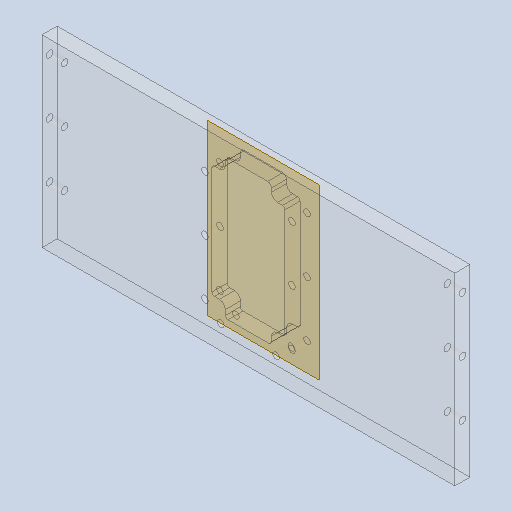
# Autodesk Inventor part: _newbody1
Saved by Autodesk Inventor 2024.3 (Build 283343000, 343)
## iProperties
Created: 2024-09-09
Part Number: _newbody1
Material: PMMA 플라스틱
Document SubType Name: Modeling
Designer: gretc
Density: 1.188 g/cm^3
Appearance: 폴리카보네이트 - 선명
Author: gretc
Autodesk Inventor part; units mm, degrees
ref_plane "YZ Plane" through (0, 0, 0) normal (1, 0, 0) x (0, 1, 0)
ref_plane "XZ Plane" through (0, 0, 0) normal (0, 1, 0) x (-1, 0, 0)
ref_plane "XY Plane" through (0, 0, 0) normal (0, 0, 1) x (1, 0, 0)
ref_plane "작업 평면1" through (0, 0, 0) normal (0, 0, 1) x (1, 0, 0)
ref_plane "작업 평면2" through (0, 0, 0) normal (0, 0, 1) x (1, 0, 0)
sketch "스케치2" plane through (0, 0, 0) normal (0, 0, 1) x (1, 0, 0)
  arc A0 (20.1, 4.5766) -> (19.5808, 6.2636) centre (17.1, 4.5766) ccw projected
  line L0 (20.1, -39.6766) -> (20.1, 4.5766) projected
  arc A1 (19.5808, -41.3636) -> (20.1, -39.6766) centre (17.1, -39.6766) ccw projected
  line L1 (15.8929, -46.7869) -> (19.5808, -41.3636) projected
  arc A2 (13.4121, -48.1) -> (15.8929, -46.7869) centre (13.4121, -45.1) ccw projected
  line L2 (-13.4121, -48.1) -> (13.4121, -48.1) projected
  arc A3 (-15.8929, -46.7869) -> (-13.4121, -48.1) centre (-13.4121, -45.1) ccw projected
  line L3 (-19.5808, -41.3636) -> (-15.8929, -46.7869) projected
  arc A4 (-20.1, -39.6766) -> (-19.5808, -41.3636) centre (-17.1, -39.6766) ccw projected
  line L4 (-20.1, 4.5766) -> (-20.1, -39.6766) projected
  arc A5 (-19.5808, 6.2636) -> (-20.1, 4.5766) centre (-17.1, 4.5766) ccw projected
  line L5 (-15.5953, 12.1246) -> (-19.5808, 6.2636) projected
  arc A6 (-13.9414, 13) -> (-15.5953, 12.1246) centre (-13.9414, 11) ccw projected
  line L6 (-7.65, 13) -> (-13.9414, 13) projected
  arc A7 (-7.65, 13) -> (-9.15, 11.5) centre (-7.65, 11.5) ccw projected
  line L7 (-9.15, 11.5) -> (-9.15, 10) projected
  arc A8 (-11.5, 7.65) -> (-9.15, 10) centre (-11.5, 10) ccw projected
  line L8 (-11.5, 7.65) -> (-13.5, 7.65) projected
  arc A9 (-13.5, 7.65) -> (-14.5, 6.65) centre (-13.5, 6.65) ccw projected
  line L9 (-14.5, 6.65) -> (-14.5, -36.15) projected
  arc A10 (-14.5, -36.15) -> (-13.5, -37.15) centre (-13.5, -36.15) ccw projected
  line L10 (-13.5, -37.15) -> (-11.5, -37.15) projected
  arc A11 (-9.15, -39.5) -> (-11.5, -37.15) centre (-11.5, -39.5) ccw projected
  line L11 (-9.15, -39.5) -> (-9.15, -41.5) projected
  arc A12 (-9.15, -41.5) -> (-8.15, -42.5) centre (-8.15, -41.5) ccw projected
  line L12 (-8.15, -42.5) -> (8.15, -42.5) projected
  arc A13 (8.15, -42.5) -> (9.15, -41.5) centre (8.15, -41.5) ccw projected
  line L13 (9.15, -41.5) -> (9.15, -39.5) projected
  arc A14 (11.5, -37.15) -> (9.15, -39.5) centre (11.5, -39.5) ccw projected
  line L14 (11.5, -37.15) -> (13.5, -37.15) projected
  arc A15 (13.5, -37.15) -> (14.5, -36.15) centre (13.5, -36.15) ccw projected
  line L15 (14.5, -36.15) -> (14.5, 6.65) projected
  arc A16 (14.5, 6.65) -> (13.5, 7.65) centre (13.5, 6.65) ccw projected
  line L16 (13.5, 7.65) -> (11.5, 7.65) projected
  arc A17 (9.15, 10) -> (11.5, 7.65) centre (11.5, 10) ccw projected
  line L17 (9.15, 10) -> (9.15, 11.5) projected
  arc A18 (9.15, 11.5) -> (7.65, 13) centre (7.65, 11.5) ccw projected
  line L18 (13.9414, 13) -> (7.65, 13) projected
  arc A19 (15.5953, 12.1246) -> (13.9414, 13) centre (13.9414, 11) ccw projected
  line L19 (19.5808, 6.2636) -> (15.5953, 12.1246) projected
  circle A20 centre (-17.3, 4) radius 1.35 projected
  circle A21 centre (-17.3, -18) radius 1.35 projected
  circle A22 centre (-11, -45.3) radius 1.35 projected
  circle A23 centre (17.3, 4) radius 1.35 projected
  circle A24 centre (17.3, -18) radius 1.35 projected
  circle A25 centre (11, -45.3) radius 1.35 projected
  circle A26 centre (-17.3, -40) radius 1.35 projected
  circle A27 centre (17.3, -40) radius 1.35 projected
  line L20 (17.3, -18) -> (-17.3, -18)
  line L21 (0, 0) -> (0, -18)
  line L22 (80, -42.5) -> (50, -42.5) projected
  line L23 (50, -42.5) -> (48, -42.5) projected
  arc A28 (44.6111, -39.875) -> (48, -42.5) centre (48, -39) ccw projected
  line L24 (44.5, -35.65) -> (44.5, 6.15) projected
  line L25 (44.5, -39) -> (44.5, -35.65) projected
  spline S0 degree 3 poles (44.6111, -39.875) (44.5897, -39.7919) (44.572, -39.711) (44.5576, -39.6325) (44.5432, -39.554) (44.532, -39.4779) (44.5235, -39.4046) (44.5149, -39.3313) (44.5091, -39.2608) (44.5053, -39.1933) (44.5016, -39.1258) (44.5, -39.0614) (44.5, -39) knots 0 0 0 0 0.25 0.25 0.25 0.5 0.5 0.5 0.75 0.75 0.75 1 1 1 1 projected
  line L26 (82, -42.5) -> (80, -42.5) projected
  line L27 (83.5, -42.5) -> (82, -42.5) projected
  arc A29 (83.5, -42.5) -> (85.5, -40.5) centre (83.5, -40.5) ccw projected
  line L28 (85.5, 11.5) -> (85.5, -40.5) projected
  line L29 (82, 17.2869) -> (82, 18.6) projected
  line L30 (79.5, 18.6) -> (82, 18.6) projected
  line L31 (77.5, 18.5993) -> (79.5, 18.5993) projected
  line L32 (77.5, 14.475) -> (77.5, 18.1607) projected
  line L33 (77.5, 18.5993) -> (77.5, 18.1607) projected
  line L34 (82, 17.2869) -> (82, 11.8636) projected
  line L35 (83.5, 13) -> (82, 13) projected
  line L36 (84, 13) -> (83.5, 13) projected
  arc A30 (85.5, 11.5) -> (84, 13) centre (84, 11.5) ccw projected
  line L37 (77.5, 13) -> (52.5, 13) projected
  line L38 (53, 17.515) -> (53, 12.415) projected
  line L39 (48, 17.2869) -> (48, 11.8636) projected
  line L40 (46.5, 13) -> (48, 13) projected
  line L41 (46, 13) -> (46.5, 13) projected
  arc A31 (46, 13) -> (44.5, 11.5) centre (46, 11.5) ccw projected
  line L42 (-80, -42.5) -> (-50, -42.5) projected
  line L43 (-85.5, -40.5) -> (-85.5, 11.5) projected
  line L44 (51, 17.515) -> (53, 17.515) projected
  line L45 (50.5, 18.5993) -> (52.5, 18.5993) projected
  line L46 (48, 18.6) -> (50.5, 18.6) projected
  line L47 (48, 18.6) -> (48, 17.2869) projected
  line L48 (52.5, 18.1607) -> (52.5, 18.5993) projected
  line L49 (52.5, 14.475) -> (52.5, 18.1607) projected
  line L50 (51, 17.515) -> (49.5, 17.515) projected
  line L51 (44.5, 6.15) -> (44.5, 10) projected
  line L52 (44.5, 10) -> (44.5, 11.5) projected
  line L53 (-83.5, 13) -> (-82, 13) projected
  line L54 (-84, 13) -> (-83.5, 13) projected
  arc A32 (-84, 13) -> (-85.5, 11.5) centre (-84, 11.5) ccw projected
  line L55 (-82, 11.8636) -> (-82, 17.2869) projected
  line L56 (-82, 18.6) -> (-82, 17.2869) projected
  line L57 (-82, 18.6) -> (-79.5, 18.6) projected
  line L58 (-77.5, 18.5993) -> (-79.5, 18.5993) projected
  line L59 (-77.5, 18.1607) -> (-77.5, 14.475) projected
  line L60 (-77.5, 18.1607) -> (-77.5, 18.5993) projected
  line L61 (-77.5, 14.475) -> (-77.5, 12.975) projected
  line L62 (-77.5, 13) -> (-52.5, 13) projected
  arc A33 (-85.5, -40.5) -> (-83.5, -42.5) centre (-83.5, -40.5) ccw projected
  line L63 (-82, -42.5) -> (-80, -42.5) projected
  line L64 (-82, -42.5) -> (-83.5, -42.5) projected
  arc A34 (-48, -42.5) -> (-44.6111, -39.875) centre (-48, -39) ccw projected
  line L65 (-50, -42.5) -> (-48, -42.5) projected
  line L66 (-44.5, 6.15) -> (-44.5, -35.65) projected
  line L67 (-44.5, -35.65) -> (-44.5, -39) projected
  spline S1 degree 3 poles (-44.5, -39) (-44.5, -39.1495) (-44.5192, -39.4463) (-44.5748, -39.7343) (-44.6111, -39.875) knots 0 0 0 0 0.5 1 1 1 1 projected
  line L68 (-44.5, 10) -> (-44.5, 6.15) projected
  line L69 (-44.5, 11.5) -> (-44.5, 10) projected
  arc A35 (-44.5, 11.5) -> (-46, 13) centre (-46, 11.5) ccw projected
  line L70 (-46, 13) -> (-46.5, 13) projected
  line L71 (-48, 17.2869) -> (-48, 11.8636) projected
  line L72 (-46.5, 13) -> (-48, 13) projected
  line L73 (-53, 12.415) -> (-53, 17.515) projected
  line L74 (-48, 17.2869) -> (-48, 18.6) projected
  line L75 (-48, 18.6) -> (-50.5, 18.6) projected
  line L76 (-50.5, 18.5993) -> (-52.5, 18.5993) projected
  line L77 (-52.5, 18.5993) -> (-52.5, 18.1607) projected
  line L78 (-52.5, 14.475) -> (-52.5, 18.1607) projected
  line L79 (-51, 17.515) -> (-53, 17.515) projected
  line L80 (-53, 12.415) -> (-53, 17.515) projected
  line L81 (-51, 12.415) -> (-51, 17.515) projected
  line L82 (-51, 12.415) -> (-53, 12.415) projected
  line L83 (-53, 12.415) -> (-53, 17.515) projected
  line L84 (-51, 17.515) -> (-53, 17.515) projected
  line L85 (13.4121, -42.5) -> (80, -42.5) projected
  line L86 (80, -42.5) -> (80, -48.5) projected
  line L87 (13.4121, -48.5) -> (80, -48.5) projected
  line L88 (13.4121, -42.5) -> (13.4121, -48.5) projected
  circle A36 centre (-11, -45.3) radius 1.35 projected
  line L89 (-48, -42.5) -> (-7.025, -42.5) projected
  line L90 (-7.025, -42.5) -> (-7.025, -48.5) projected
  line L91 (-48, -48.5) -> (-7.025, -48.5) projected
  line L92 (-48, -42.5) -> (-48, -48.5) projected
  line L93 (-80, -42.5) -> (-50, -42.5) projected
  line L94 (-50, -42.5) -> (-50, -48.5) projected
  line L95 (-80, -48.5) -> (-50, -48.5) projected
  line L96 (-80, -42.5) -> (-80, -48.5) projected
  line L97 (-50, -42.5) -> (-48, -42.5) projected
  line L98 (-48, -42.5) -> (-48, -48.5) projected
  line L99 (-50, -48.5) -> (-48, -48.5) projected
  line L100 (-50, -42.5) -> (-50, -48.5) projected
  line L101 (-82, -42.5) -> (-80, -42.5) projected
  line L102 (-80, -42.5) -> (-80, -48.5) projected
  line L103 (-82, -48.5) -> (-80, -48.5) projected
  line L104 (-82, -42.5) -> (-82, -48.5) projected
  line L105 (82, -54.5993) -> (82, 18.5993)
  line L106 (82, 18.5993) -> (-82, 18.5993)
  line L107 (-82, 18.5993) -> (-82, -54.5993)
  line L108 (-82, -54.5993) -> (82, -54.5993)
  line L109 (82, -54.5993) -> (-82, 18.5993) construction
  line L110 (82, 18.5993) -> (-82, -54.5993) construction
  line L111 (7.65, 13) -> (-7.65, 13)
  line L112 (-7.65, 13) -> (-7.65, 18.5993)
  line L113 (-7.65, 18.5993) -> (7.65, 18.5993)
  line L114 (7.65, 18.5993) -> (7.65, 13)
  point P0 (77.5, 12.975)
  point P1 (82, 18.5993)
  constraints: 24 end point, 4 parallel, 3 midpoint, 2 horizontal, 2 perpendicular, 1 coincident, 1 vertical, 1 other
extrude "돌출1" add sketch "스케치2" along normal blind 6 contours L0 A1 L1 L85 L88 L2 L90 L12 A13 L13 A14 L14 A15 L15 A16 L16 A17 L17 A18 L18 A19 L19 A0 | A0 L19 A19 L18 L114 L106 L47 L39 L40 L41 A31 L52 L51 L24 L25 S0 A28 L85 L1 A1 L0 | L85 L23 L22 L86 L87 L88 A2 L1 | L1 A2 L88 L85 | L111 L112 L106 L114 | A28 S0 L25 L24 L51 L52 A31 L41 L40 L39 L47 L46 L45 L106 L31 L30 L29 L34 L105 L26 L22 L23 | A7 L7 A8 L8 A9 L9 A10 L10 A11 L11 A12 L89 L3 A4 L4 A5 L5 A6 L6 | L6 A6 L5 A5 L4 A4 L3 L89 A34 S1 L67 L66 L68 L69 A35 L70 L72 L71 L74 L106 L112 | L88 L87 L86 L26 L105 L108 L107 L103 L95 L99 L91 L90 L2 | L90 L91 L92 L89 L3 A3 L2 | L2 A3 L3 L89 L12 L90 | L74 L71 L72 L70 A35 L69 L68 L66 L67 S1 A34 L65 L42 L63 L107 L55 L56 L57 L58 L60 L59 L61 L62 L73 L82 L81 L79 L78 L77 L76 L75 | L99 L94 L65 L92 | L77 L78 L79 L73 L62 L61 L59 L60 L106 | L95 L96 L42 L94 | L103 L104 L63 L96 | L79 L81 L82 L73
sketch "스케치3" plane through (82, -54.5993, 0) normal (1, 0, 0) x (0, 0, -1)
  circle A0 centre (-3, 65.0993) radius 1.35 projected
  circle A1 centre (-3, 43.0993) radius 1.35 projected
  circle A2 centre (-3, 21.0993) radius 1.35 projected
  point P0 (0, 54.5993)
extrude "돌출2" cut sketch "스케치3" against normal blind 6
sketch "스케치4" plane through (-82, -54.5993, 0) normal (-1, 0, 0) x (0, 0, 1)
  circle A0 centre (3, 65.0993) radius 1.35 projected
  circle A1 centre (3, 43.0993) radius 1.35 projected
  circle A2 centre (3, 21.0993) radius 1.35 projected
  point P0 (0, 54.5993)
extrude "돌출3" cut sketch "스케치4" against normal blind 6
